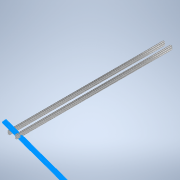
# Autodesk Inventor part: 2040 ext 1800
Saved by Autodesk Inventor 2020 (Build 240168000, 168)
## iProperties
Created: 2020-07-11
Part Number: 2040 ext 1800
Material: Generic
Document SubType Name: Modeling
Designer: Vikki
Density: 1 g/cm^3
Appearance: Chrome - Polished
Author: Vikki
Autodesk Inventor part; units mm, degrees
ref_plane "YZ Plane" through (0, 0, 0) normal (1, 0, 0) x (0, 1, 0)
ref_plane "XZ Plane" through (0, 0, 0) normal (0, 1, 0) x (-1, 0, 0)
ref_plane "XY Plane" through (0, 0, 0) normal (0, 0, 1) x (1, 0, 0)
sketch "Sketch1" plane through (0, 0, 0) normal (0, 0, 1) x (1, 0, 0)
  arc A0 (10, 18.5) -> (8.5, 20) centre (8.5, 18.5) ccw projected
  line L0 (10, 18.5) -> (10, 13.6) projected
  line L1 (10, 13.6) -> (9.3, 13.6) projected
  arc A1 (9.3, 13.6) -> (9.1, 13.4) centre (9.3, 13.4) ccw projected
  line L2 (9.1, 13.4) -> (9.1, 13.1) projected
  line L3 (9.1, 13.1) -> (8.2, 13.1) projected
  line L4 (8.2, 13.1) -> (8.2, 15.45) projected
  line L5 (8.2, 15.45) -> (6.2985, 15.45) projected
  line L6 (6.2985, 15.45) -> (3.9, 13.0515) projected
  line L7 (3.9, 13.0515) -> (3.9, 6.9485) projected
  line L8 (3.9, 6.9485) -> (6.2985, 4.55) projected
  line L9 (6.2985, 4.55) -> (8.2, 4.55) projected
  line L10 (8.2, 4.55) -> (8.2, 6.9) projected
  line L11 (8.2, 6.9) -> (9.1, 6.9) projected
  line L12 (9.1, 6.9) -> (9.1, 6.6) projected
  arc A2 (9.1, 6.6) -> (9.3, 6.4) centre (9.3, 6.6) ccw projected
  line L13 (9.3, 6.4) -> (10, 6.4) projected
  line L14 (10, 6.4) -> (10, -6.4) projected
  line L15 (10, -6.4) -> (9.3, -6.4) projected
  arc A3 (9.3, -6.4) -> (9.1, -6.6) centre (9.3, -6.6) ccw projected
  line L16 (9.1, -6.6) -> (9.1, -6.9) projected
  line L17 (9.1, -6.9) -> (8.2, -6.9) projected
  line L18 (8.2, -6.9) -> (8.2, -4.55) projected
  line L19 (8.2, -4.55) -> (6.2985, -4.55) projected
  line L20 (6.2985, -4.55) -> (3.9, -6.9485) projected
  line L21 (3.9, -6.9485) -> (3.9, -13.0515) projected
  line L22 (3.9, -13.0515) -> (6.2985, -15.45) projected
  line L23 (6.2985, -15.45) -> (8.2, -15.45) projected
  line L24 (8.2, -15.45) -> (8.2, -13.1) projected
  line L25 (8.2, -13.1) -> (9.1, -13.1) projected
  line L26 (9.1, -13.1) -> (9.1, -13.4) projected
  arc A4 (9.1, -13.4) -> (9.3, -13.6) centre (9.3, -13.4) ccw projected
  line L27 (9.3, -13.6) -> (10, -13.6) projected
  line L28 (10, -13.6) -> (10, -18.5) projected
  arc A5 (8.5, -20) -> (10, -18.5) centre (8.5, -18.5) ccw projected
  line L29 (8.5, -20) -> (3.6, -20) projected
  line L30 (3.6, -20) -> (3.6, -19.3) projected
  arc A6 (3.6, -19.3) -> (3.4, -19.1) centre (3.4, -19.3) ccw projected
  line L31 (3.4, -19.1) -> (3.1, -19.1) projected
  line L32 (3.1, -19.1) -> (3.1, -18.2) projected
  line L33 (3.1, -18.2) -> (5.45, -18.2) projected
  line L34 (5.45, -18.2) -> (5.45, -16.2985) projected
  line L35 (5.45, -16.2985) -> (3.0515, -13.9) projected
  line L36 (3.0515, -13.9) -> (-3.0515, -13.9) projected
  line L37 (-3.0515, -13.9) -> (-5.45, -16.2985) projected
  line L38 (-5.45, -16.2985) -> (-5.45, -18.2) projected
  line L39 (-5.45, -18.2) -> (-3.1, -18.2) projected
  line L40 (-3.1, -18.2) -> (-3.1, -19.1) projected
  line L41 (-3.1, -19.1) -> (-3.4, -19.1) projected
  arc A7 (-3.4, -19.1) -> (-3.6, -19.3) centre (-3.4, -19.3) ccw projected
  line L42 (-3.6, -19.3) -> (-3.6, -20) projected
  line L43 (-3.6, -20) -> (-8.5, -20) projected
  arc A8 (-10, -18.5) -> (-8.5, -20) centre (-8.5, -18.5) ccw projected
  line L44 (-10, -18.5) -> (-10, -13.6) projected
  line L45 (-10, -13.6) -> (-9.3, -13.6) projected
  arc A9 (-9.3, -13.6) -> (-9.1, -13.4) centre (-9.3, -13.4) ccw projected
  line L46 (-9.1, -13.4) -> (-9.1, -13.1) projected
  line L47 (-9.1, -13.1) -> (-8.2, -13.1) projected
  line L48 (-8.2, -13.1) -> (-8.2, -15.45) projected
  line L49 (-8.2, -15.45) -> (-6.2985, -15.45) projected
  line L50 (-6.2985, -15.45) -> (-3.9485, -13.1) projected
  line L51 (-3.9485, -13.1) -> (-3.9485, -6.9) projected
  line L52 (-3.9485, -6.9) -> (-6.2985, -4.55) projected
  line L53 (-6.2985, -4.55) -> (-8.2, -4.55) projected
  line L54 (-8.2, -4.55) -> (-8.2, -6.9) projected
  line L55 (-8.2, -6.9) -> (-9.1, -6.9) projected
  line L56 (-9.1, -6.9) -> (-9.1, -6.6) projected
  arc A10 (-9.1, -6.6) -> (-9.3, -6.4) centre (-9.3, -6.6) ccw projected
  line L57 (-9.3, -6.4) -> (-10, -6.4) projected
  line L58 (-10, -6.4) -> (-10, 6.4) projected
  line L59 (-10, 6.4) -> (-9.3, 6.4) projected
  arc A11 (-9.3, 6.4) -> (-9.1, 6.6) centre (-9.3, 6.6) ccw projected
  line L60 (-9.1, 6.6) -> (-9.1, 6.9) projected
  line L61 (-9.1, 6.9) -> (-8.2, 6.9) projected
  line L62 (-8.2, 6.9) -> (-8.2, 4.55) projected
  line L63 (-8.2, 4.55) -> (-6.2985, 4.55) projected
  line L64 (-6.2985, 4.55) -> (-3.9485, 6.9) projected
  line L65 (-3.9485, 6.9) -> (-3.9485, 13.1) projected
  line L66 (-3.9485, 13.1) -> (-6.2985, 15.45) projected
  line L67 (-6.2985, 15.45) -> (-8.2, 15.45) projected
  line L68 (-8.2, 15.45) -> (-8.2, 13.1) projected
  line L69 (-8.2, 13.1) -> (-9.1, 13.1) projected
  line L70 (-9.1, 13.1) -> (-9.1, 13.4) projected
  arc A12 (-9.1, 13.4) -> (-9.3, 13.6) centre (-9.3, 13.4) ccw projected
  line L71 (-9.3, 13.6) -> (-10, 13.6) projected
  line L72 (-10, 13.6) -> (-10, 18.5) projected
  arc A13 (-8.5, 20) -> (-10, 18.5) centre (-8.5, 18.5) ccw projected
  line L73 (-8.5, 20) -> (-3.6, 20) projected
  line L74 (-3.6, 20) -> (-3.6, 19.3) projected
  arc A14 (-3.6, 19.3) -> (-3.4, 19.1) centre (-3.4, 19.3) ccw projected
  line L75 (-3.4, 19.1) -> (-3.1, 19.1) projected
  line L76 (-3.1, 19.1) -> (-3.1, 18.2) projected
  line L77 (-3.1, 18.2) -> (-5.45, 18.2) projected
  line L78 (-5.45, 18.2) -> (-5.45, 16.2985) projected
  line L79 (-5.45, 16.2985) -> (-3.0515, 13.9) projected
  line L80 (-3.0515, 13.9) -> (3.0515, 13.9) projected
  line L81 (3.0515, 13.9) -> (5.45, 16.2985) projected
  line L82 (5.45, 16.2985) -> (5.45, 18.2) projected
  line L83 (5.45, 18.2) -> (3.1, 18.2) projected
  line L84 (3.1, 18.2) -> (3.1, 19.1) projected
  line L85 (3.1, 19.1) -> (3.4, 19.1) projected
  arc A15 (3.4, 19.1) -> (3.6, 19.3) centre (3.4, 19.3) ccw projected
  line L86 (3.6, 19.3) -> (3.6, 20) projected
  line L87 (3.6, 20) -> (8.5, 20) projected
  line L88 (5.8015, -3.35) -> (8.2, -3.35) projected
  line L89 (8.2, -3.35) -> (8.2, 3.35) projected
  line L90 (8.2, 3.35) -> (5.8015, 3.35) projected
  line L91 (5.8015, 3.35) -> (3.0515, 6.1) projected
  line L92 (3.0515, 6.1) -> (-3.0515, 6.1) projected
  line L93 (-3.0515, 6.1) -> (-5.8015, 3.35) projected
  line L94 (-5.8015, 3.35) -> (-8.2, 3.35) projected
  line L95 (-8.2, 3.35) -> (-8.2, -3.35) projected
  line L96 (-8.2, -3.35) -> (-5.8015, -3.35) projected
  line L97 (-5.8015, -3.35) -> (-3.0515, -6.1) projected
  line L98 (-3.0515, -6.1) -> (3.0515, -6.1) projected
  line L99 (3.0515, -6.1) -> (5.8015, -3.35) projected
  circle A16 centre (0, 10) radius 2.5 projected
  circle A17 centre (0, -10) radius 2.5 projected
  point P0 (0, 0)
extrude "Extrusion1" add sketch "Sketch1" against normal blind 1700
pattern_linear "Rectangular Pattern1" count 2 spacing 80 along (-1, 0, 0) of "Extrusion1"
body "Solid1"
